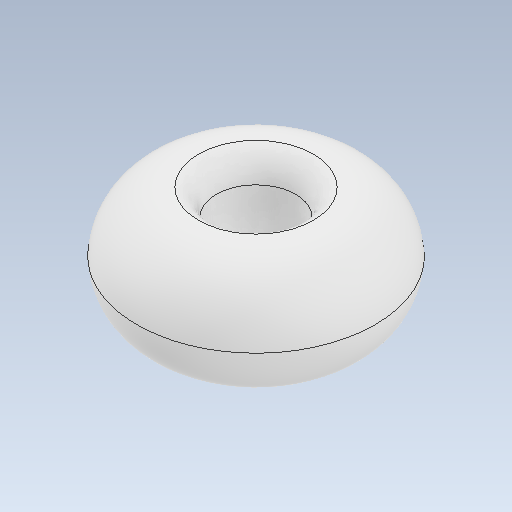
# Autodesk Inventor part: 8000_132uH_DCore_2layer_Tx_Filter_MPSv2_v1
Saved by Autodesk Inventor 2021 (Build 250183000, 183)
## iProperties
Created: 2020-12-10
Part Number: 8000_132uH_DCore_2layer_Tx_Filter_MPSv2_v1
Material: ABS Plastic
Document SubType Name: Modeling
Designer: Barksdale
Density: 1.06 g/cm^3
Appearance: Smooth - White
Author: Barksdale
Autodesk Inventor part; units mm, degrees
ref_plane "YZ Plane" through (0, 0, 0) normal (1, 0, 0) x (0, 1, 0)
ref_plane "XZ Plane" through (0, 0, 0) normal (0, 1, 0) x (-1, 0, 0)
ref_plane "XY Plane" through (0, 0, 0) normal (0, 0, 1) x (1, 0, 0)
sketch "Sketch1" plane through (0, 0, 0) normal (0, 0, 1) x (1, 0, 0)
  line L0 (0, 0) -> (10.4, 0)
  line L1 (0, 0) -> (31.2, 0)
  line L2 (0, 0) -> (22.1, 0)
  line L3 (10.4, 0) -> (28.4, 0)
  line L4 (0, 0) -> (18, 0)
  line L5 (10.4, 0) -> (10.4, 8.8)
  arc A0 (15.0348, 15.6) -> (10.4, 8.8) centre (17.9974, 8.6012) ccw
  line L6 (18, 0) -> (18, 15.6)
  line L7 (18, 15.6) -> (15.0348, 15.6)
  arc A1 (31.2, 0) -> (15.0348, 15.6) centre (15.0348, -0.5755) ccw
  line L8 (10.4, 0) -> (10.4, -8.8)
  arc A2 (10.4, -8.8) -> (15.0348, -15.6) centre (17.9974, -8.6012) ccw
  arc A3 (15.0348, -15.6) -> (31.2, 0) centre (15.0348, 0.5755) ccw
  line L9 (0, 0) -> (0, 15.6)
  dimension "d0" = 10.4
  dimension "d1" = 31.2
  dimension "d4" = 18
  dimension "d5" = 8.8
  dimension "d6" = 15.6
  constraints: 20 end point, 8 point on circle, 4 centre point, 4 symmetric about line, 3 point on line, 2 horizontal, 2 perpendicular, 2 vertical, 1 tangent, 2 other
  measures "d0" distance of L0.start L0.end
  measures "d1" distance of L0.start L1.end
  measures "d4" distance of L0.start L4.end
  measures "d5" distance of L5.end L0.end
  measures "d6" distance of L4.end L6.end
revolve "Revolution1" add sketch "Sketch1" angle 360 about axis through (0, 0, 0) along (0, -1, 0) contours L5 A0 A1 L6 L1 | L1 A3 A2 L8 | L6 A1 L1
body "Solid1"
